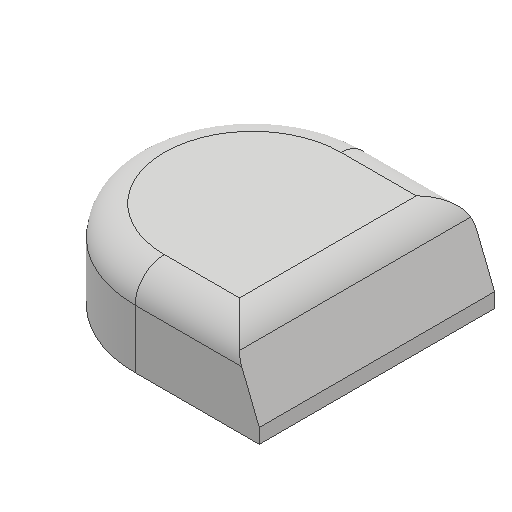
# Autodesk Inventor part: 3DP_ABS_Front_Door_Magnet_Holder
Saved by Autodesk Inventor 2026.1 (Build 301233000, 233)
## iProperties
Created: 2016-06-28
Part Number: 3DP_ABS_Front_Door_Magnet_Holder
Material: Ogólny
Document SubType Name: Modeling
Designer: Andrzej
Density: 1 g/cm^3
Appearance: Domyślna
Author: Andrzej
Autodesk Inventor part; units mm, degrees
ref_plane "YZ Plane" through (0, 0, 0) normal (1, 0, 0) x (0, 1, 0)
ref_plane "XZ Plane" through (0, 0, 0) normal (0, 1, 0) x (-1, 0, 0)
ref_plane "XY Plane" through (0, 0, 0) normal (0, 0, 1) x (1, 0, 0)
sketch "Szkic1" plane through (0, 0, 0) normal (0, 0, 1) x (1, 0, 0)
  line L0 (0, 6.5573) -> (0, -9.5427)
  circle A0 centre (-8.5, -1.4927) radius 5.05
  arc A1 (-8.5, 6.5573) -> (-8.5, -9.5427) centre (-8.5, -1.4927) ccw
  line L1 (0, 6.5573) -> (-8.5, 6.5573)
  line L2 (0, -9.5427) -> (-8.5, -9.5427)
  point P0 (0, 0)
  dimension "d0" = 16.1
  dimension "d1" = 8.5
  dimension "d2" = 10.1
  dimension "d3" = 8.05
  dimension "d4" = 3
  constraints: 6 end point, 2 centre point, 2 point on circle, 2 tangent, 1 coincident, 1 vertical
  measures "d0" distance of L0.start L0.end
  measures "d1" distance from line of L0 point (-8.5, -1.493)
  measures "d2" diameter of A0
  measures "d3" vertical distance of A0.centre L0.start
  measures "d4" radial gap between concentric circles of A0 A1
extrude "Wyciągnięcie proste1" add sketch "Szkic1" along normal blind 6 contours L0 L2 A1 L1 | A0
chamfer "Faza1" distance 2 distance2 5 1 edges at (0, -1.4927, 6) measured on face at (-2.8333, -4.176, 6)
extrude "Wyciągnięcie proste2" cut sketch "Szkic1" along normal blind 4.25 contours A0
fillet "Zaokrąglenie1" radius 2 4 edges at (-16.55, -1.4927, 6) (-5.25, -9.5427, 6) (-5.25, 6.5573, 6) (-2, -1.4927, 6)
equation "\"d3\" = 0.5 * d0"
